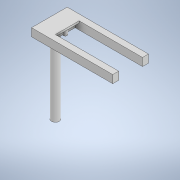
# Autodesk Inventor part: ServoHållare
Saved by Autodesk Inventor 2021 (Build 250183000, 183)
## iProperties
Created: 2024-03-20
Part Number: ServoHållare
Material: Generic
Document SubType Name: Modeling
Designer: 21seblin
Density: 1 g/cm^3
Appearance: Default
Author: 21seblin
Autodesk Inventor part; units mm, degrees
ref_plane "YZ Plane" through (0, 0, 0) normal (1, 0, 0) x (0, 1, 0)
ref_plane "XZ Plane" through (0, 0, 0) normal (0, 1, 0) x (-1, 0, 0)
ref_plane "XY Plane" through (0, 0, 0) normal (0, 0, 1) x (1, 0, 0)
sketch "Sketch1" plane through (0, 0, 0) normal (0, 1, 0) x (-1, 0, 0)
  line L0 (18, 9) -> (-18, 9)
  line L1 (-18, 9) -> (-18, -9)
  line L2 (-18, -9) -> (18, -9)
  line L3 (18, -9) -> (18, 9)
  line L4 (18, 9) -> (-18, -9) construction
  line L5 (-18, 9) -> (18, -9) construction
  point P0 (0, 0)
  dimension "d0" = 18
  dimension "d1" = 36
  constraints: 12 end point, 2 midpoint, 2 parallel, 1 horizontal, 1 perpendicular
  measures "d0" distance of L0.end L1.end
  measures "d1" distance of L1.end L2.end
extrude "Extrusion1" add sketch "Sketch1" along normal blind 4
sketch "Sketch2" plane through (18, 0, 9) normal (1, 0, 0) x (0, 0, -1)
  line L0 (3, 9.8571) -> (15, 9.8571)
  line L1 (15, 9.8571) -> (15, 0)
  line L2 (15, 0) -> (3, 0)
  line L3 (3, 0) -> (3, 9.8571)
  line L4 (0.7991, 7.2165) -> (12.7991, -2.6406) construction
  line L5 (12.7991, 7.2165) -> (0.7991, -2.6406) construction
  line L6 (9, 0) -> (9, 4.0958)
  line L7 (9, 0) -> (15, 0)
  line L8 (0, 0) -> (18, 0) projected
  point P0 (6.7991, 2.2879)
  dimension "d4" = 12
  dimension "d22" = 6
  constraints: 16 end point, 2 midpoint, 2 parallel, 2 point on line, 1 horizontal, 1 perpendicular, 1 vertical
  measures "d4" distance of L1.end L2.end
  measures "d22" distance of L6.start L7.end
extrude "Extrusion2" cut sketch "Sketch2" against normal blind 34
sketch "Sketch3" plane through (-16, 0, 9) normal (1, 0, 0) x (0, 0, -1)
  line L0 (3, 4) -> (15, 4) projected
  line L1 (15, 4) -> (15, 0) projected
  line L2 (3, 4) -> (15, 4)
  line L3 (15, 4) -> (15, 3)
  line L4 (15, 3) -> (3, 3)
  line L5 (3, 3) -> (3, 4)
  point P0 (9, 0)
  dimension "d7" = 1
  constraints: 8 end point, 2 parallel, 1 horizontal, 1 perpendicular, 1 point on line
  measures "d7" distance of L3.end L2.end
extrude "Extrusion3" add sketch "Sketch3" along normal blind 2
sketch "Sketch4" plane through (-16, 3, -6) normal (0, -1, 0) x (1, 0, 0)
  line L0 (0, 12) -> (2, 12) projected
  line L1 (1, 12) -> (1, 0)
  line L2 (2, 0) -> (0, 0) projected
  line L3 (2, 0) -> (2, 12) projected
  line L4 (2, 6) -> (0, 6)
  line L5 (0, 0) -> (0, 12) projected
  circle A0 centre (1, 6) radius 0.95
  point P0 (16, 6)
  dimension "d10" = 1.9
  constraints: 5 midpoint, 4 end point, 1 centre point
  measures "d10" diameter of A0
extrude "Extrusion4" add sketch "Sketch4" along normal blind 2.5 contours A0 L4 L1 | L1 L4 A0 | L4 L1 A0 | L4 A0 L1
sketch "Sketch5" plane through (-18, 0, -9) normal (-1, 0, 0) x (0, 0, 1)
  line L0 (18, 0) -> (15, 0) projected
  line L1 (0, 0) -> (0, 4) projected
  line L2 (18, 0) -> (0, 0)
  line L3 (0, 0) -> (0, 1)
  line L4 (0, 1) -> (18, 1)
  line L5 (18, 1) -> (18, 0)
  point P0 (9, 0)
  dimension "d13" = 1
  constraints: 8 end point, 2 parallel, 1 horizontal, 1 perpendicular, 1 point on line
  measures "d13" distance of L4.end L0.start
extrude "Extrusion5" add sketch "Sketch5" along normal blind 5
sketch "Sketch6" plane through (-18, 1, 9) normal (0, 1, 0) x (1, 0, 0)
  line L0 (0, 18) -> (0, 0) projected
  line L1 (0, 9) -> (-2, 9)
  circle A0 centre (-2, 9) radius 1.95
  point P0 (18, 9)
  dimension "d16" = 2
  dimension "d17" = 3.9
  constraints: 2 end point, 1 centre point, 1 coincident, 1 horizontal, 1 midpoint
  measures "d16" distance of L1.start L1.end
  measures "d17" diameter of A0
extrude "Extrusion6" add sketch "Sketch6" against normal blind 40
sketch "Sketch7" plane through (-18, 1, 9) normal (0, 1, 0) x (1, 0, 0)
  line L0 (0, 0) -> (-5, 0) projected
  line L1 (-5, 18) -> (-5, 0) projected
  line L2 (0, 0) -> (-5, 0)
  line L3 (-5, 0) -> (-5, 18)
  line L4 (-5, 18) -> (0, 18)
  line L5 (0, 18) -> (0, 0)
  point P0 (18, 9)
  constraints: 8 end point, 2 parallel, 1 horizontal, 1 perpendicular
extrude "Extrusion7" add sketch "Sketch7" along normal blind 3
body "Solid1"
